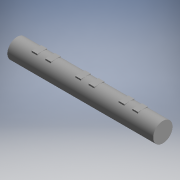
# Autodesk Inventor part: Eje
Saved by Autodesk Inventor 2019.3 (Build 233278000, 278)
## iProperties
Part Number: Eje
Material: Generic
Document SubType Name: Modeling
Designer: Usuario
Appearance: Default
Author: Usuario
Autodesk Inventor part; units mm, degrees
ref_plane "YZ Plane" through (0, 0, 0) normal (1, 0, 0) x (0, 1, 0)
ref_plane "XZ Plane" through (0, 0, 0) normal (0, 1, 0) x (-1, 0, 0)
ref_plane "XY Plane" through (0, 0, 0) normal (0, 0, 1) x (1, 0, 0)
sketch "Sketch1" plane through (0, 0, 0) normal (0, 0, 1) x (1, 0, 0)
  line L0 (0, 0) -> (381, 0)
  line L1 (0, 0) -> (0, 25.4)
  line L2 (0, 25.4) -> (50.8, 25.4)
  line L3 (50.8, 25.4) -> (50.8, 28.575)
  line L4 (50.8, 28.575) -> (65.786, 28.575)
  line L5 (65.786, 28.575) -> (65.786, 25.4)
  line L6 (65.786, 25.4) -> (86.106, 25.4)
  line L7 (86.106, 25.4) -> (86.106, 28.575)
  line L8 (86.106, 28.575) -> (101.092, 28.575)
  line L9 (101.092, 28.575) -> (101.092, 25.4)
  line L10 (101.092, 25.4) -> (164.592, 25.4)
  line L11 (164.592, 28.575) -> (179.578, 28.575)
  line L12 (179.578, 28.575) -> (179.578, 25.4)
  line L13 (179.578, 25.4) -> (199.898, 25.4)
  line L14 (199.898, 25.4) -> (199.898, 28.575)
  line L15 (199.898, 28.575) -> (214.884, 28.575)
  line L16 (214.884, 28.575) -> (214.884, 25.4)
  line L17 (214.884, 25.4) -> (278.384, 25.4)
  line L18 (278.384, 28.575) -> (293.37, 28.575)
  line L19 (293.37, 28.575) -> (293.37, 25.4)
  line L20 (293.37, 25.4) -> (313.69, 25.4)
  line L21 (313.69, 25.4) -> (313.69, 28.575)
  line L22 (313.69, 28.575) -> (328.676, 28.575)
  line L23 (328.676, 28.575) -> (328.676, 25.4)
  line L24 (328.676, 25.4) -> (379.476, 25.4)
  line L25 (164.592, 28.575) -> (164.592, 25.4)
  line L26 (278.384, 28.575) -> (278.384, 25.4)
  line L27 (379.476, 25.4) -> (381, 25.4)
  line L28 (381, 25.4) -> (381, 0)
  dimension "d0" = 381
  dimension "d1" = 25.4
  dimension "d2" = 50.8
  dimension "d3" = 3.175
  dimension "d4" = 14.986
  dimension "d5" = 20.32
  dimension "d6" = 14.986
  dimension "d7" = 63.5
  dimension "d8" = 14.986
  dimension "d9" = 20.32
  dimension "d10" = 14.986
  dimension "d11" = 63.5
  dimension "d12" = 14.986
  dimension "d13" = 20.32
  dimension "d14" = 14.986
  dimension "d15" = 50.8
  constraints: 58 end point, 14 point on line, 13 perpendicular, 2 horizontal, 2 vertical, 1 parallel
  measures "d0" distance of L0.start L0.end
  measures "d1" distance of L0.start L1.end
  measures "d2" distance of L1.end L2.end
  measures "d3" distance of L2.end L3.end
  measures "d4" distance of L3.end L4.end
  measures "d5" distance of L5.end L6.end
  measures "d6" distance of L7.end L8.end
  measures "d7" distance of L9.end L10.end
  measures "d8" distance of L11.start L11.end
  measures "d9" distance of L12.end L13.end
  measures "d10" distance of L14.end L15.end
  measures "d11" distance of L16.end L17.end
  measures "d12" distance of L18.start L18.end
  measures "d13" distance of L19.end L20.end
  measures "d14" distance of L21.end L22.end
  measures "d15" distance of L23.end L24.end
revolve "Revolution1" add sketch "Sketch1" angle 360 about axis through (0, 0, 0) along (1, 0, 0)
sketch "Sketch2" plane through (381, 0, 0) normal (1, 0, 0) x (0, 0, -1)
  circle A0 centre (0, 0) radius 28.575
  arc A1 (-12.8501, 21.8127) -> (12.8501, 21.9887) centre (0.1501, -0.0084) ccw
  line L0 (28.575, -0.0084) -> (28.6569, -0.0084) construction
  line L1 (28.5738, -0.2635) -> (28.6458, -0.2635) construction
  line L2 (12.8501, 21.9887) -> (12.8501, 25.5227)
  line L3 (-12.8501, 21.8127) -> (-12.8501, 25.5227)
  line L4 (12.8501, 25.5227) -> (-12.8501, 25.5227)
  constraints: 10 end point, 6 point on circle, 2 centre point, 2 horizontal, 2 vertical, 1 perpendicular
sketch "Sketch3" plane through (0, 0, 0) normal (-1, 0, 0) x (0, 0, 1)
  circle A0 centre (0, 0) radius 28.575
  arc A1 (-12.7, 21.997) -> (12.7, 21.997) centre (0, 0) ccw
  circle A2 centre (0, 0) radius 28.575 projected
  line L0 (-12.7, 21.997) -> (-12.7, 25.5977)
  line L1 (12.7, 21.997) -> (12.7, 25.5977)
  line L2 (-12.7, 25.5977) -> (12.7, 25.5977)
  dimension "d23" = 57.15
  dimension "d24" = 50.8
  constraints: 6 end point, 2 centre point, 2 coincident, 2 point on circle, 2 vertical, 3 other
  measures "d23" diameter of A0
  measures "d24" diameter of A1
extrude "Extrusion1" cut sketch "Sketch3" against normal blind 381 contours A0 L0 A1 L1 | L2 A0
body "Solid1"
